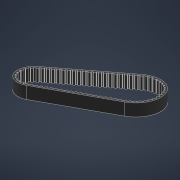
# Autodesk Inventor part: Parametric GT2 Belt v1
Saved by Autodesk Inventor 2021 (Build 250183000, 183)
## iProperties
Created: 2020-06-05
Part Number: Parametric GT2 Belt v1
Material: Rubber
Document SubType Name: Modeling
Designer: Bryce
Density: 0.93 g/cm^3
Appearance: Rubber - Black
Author: Bryce
Autodesk Inventor part; units mm, degrees
ref_plane "YZ Plane" through (0, 0, 0) normal (1, 0, 0) x (0, 1, 0)
ref_plane "XY Plane" through (0, 0, 0) normal (0, 0, 1) x (1, 0, 0)
sketch "top teeth placement" plane through (0, 0, 0) normal (0, 1, 0) x (-1, 0, 0)
  arc A0 (1.0993, -11.4063) -> (1.0993, 11.4063) centre (0, 0) ccw construction
  line L0 (1.0993, -11.4063) -> (-58.0762, -17.1095) construction
  line L1 (1.0993, 11.4063) -> (-58.0762, 17.1095) construction
  arc A1 (-58.0762, 17.1095) -> (-58.0762, -17.1095) centre (-59.7252, 0) ccw construction
  arc A2 (1.0993, -11.4063) -> (4.014, -10.7331) centre (0, 0) ccw construction
  arc A3 (-61.6201, -17.084) -> (-58.0762, -17.1095) centre (-59.7252, 0) ccw construction
  arc A4 (-64.5579, -16.4954) -> (-61.6201, -17.084) centre (-59.7252, 0) ccw construction
  line L2 (1.0993, -11.4063) -> (0, 0) construction
  line L3 (0, 0) -> (4.014, -10.7331) construction
  line L4 (-61.6201, -17.084) -> (-59.7252, 0) construction
  line L5 (-59.7252, 0) -> (-64.5579, -16.4954) construction
  point P0 (-1.8869, -11.6941)
  point P1 (-4.873, -11.9819)
  point P2 (-7.8592, -12.2697)
  point P3 (-10.8454, -12.5575)
  point P4 (-13.8315, -12.8453)
  point P5 (-16.8177, -13.1331)
  point P6 (-1.0925, 11.6175)
  point P7 (-4.0787, 11.9053)
  point P8 (-19.8038, -13.4209)
  point P9 (-22.79, -13.7087)
  point P10 (-25.7762, -13.9965)
  point P11 (-28.7623, -14.2843)
  point P12 (-31.7485, -14.5721)
  point P13 (-34.7347, -14.8599)
  point P14 (-37.7208, -15.1477)
  point P15 (-40.707, -15.4355)
  point P16 (-43.6931, -15.7233)
  point P17 (-46.6793, -16.0111)
  point P18 (-49.6655, -16.2989)
  point P19 (-52.6516, -16.5867)
  point P20 (-55.6378, -16.8745)
  point P21 (-58.624, -17.1622)
  dimension "pitch" = 3
  dimension "r_d35" = 60
  dimension "r_d36" = 33
  dimension "d17" = 22.9183
  dimension "d18" = 34.3775
  dimension "d30" = 3
  dimension "d35" = 59.4497
  dimension "d36" = 33.798
  dimension "d39" = 15
  dimension "d41" = 3
  dimension "d44" = 3.5503
  dimension "d45" = 57.303
  dimension "d48" = 10
  dimension "d50" = 3
  dimension "d52" = 2.202
  dimension "d62" = 3
  dimension "d71" = 59.7252
  constraints: 12 end point, 11 point on circle, 5 centre point, 4 coincident, 4 tangent, 3 concentric, 1 horizontal alignment, 1 point on line, 27 other
  measures "d17" diameter of A0
  measures "d18" diameter of A1
  measures "d30" distance of L2.start point (-1.887, -11.694)
  measures "d35" distance of L0.start L0.end
  measures "d52" distance of point (-1.093, 11.618) L1.start
  measures "d62" distance of point (-1.093, 11.618) point (-4.079, 11.905)
  measures "d71" distance of A1.centre point (0, 0)
sketch "gt2 profile" plane through (0, 0, 0) normal (0, 1, 0) x (-1, 0, 0)
  line L0 (-61.6201, -17.084) -> (-59.7252, 0) construction
  arc A0 (-58.0762, 17.1095) -> (-58.0762, -17.1095) centre (-59.7252, 0) ccw construction
  line L1 (1.0993, -11.4063) -> (-58.0762, -17.1095) construction
  line L2 (1.0993, 11.4063) -> (-58.0762, 17.1095) construction
  arc A1 (1.787, -10.3422) -> (0.2211, -10.4931) centre (1.0349, -10.7384) ccw
  arc A2 (1.9264, -10.723) -> (2.1945, -10.918) centre (2.1705, -10.6691) ccw
  line L3 (2.1945, -10.918) -> (-0.069, -11.1361)
  line L4 (0.4422, -11.0507) -> (1.0593, -10.9912) construction
  arc A3 (1.9264, -10.723) -> (1.787, -10.3422) centre (0.4422, -11.0507) ccw
  arc A4 (-0.069, -11.1361) -> (0.1569, -10.8936) centre (-0.093, -10.8873) ccw
  arc A5 (0.2211, -10.4931) -> (0.1569, -10.8936) centre (1.6764, -10.9317) ccw
  line L5 (2.2905, -11.9134) -> (0.0269, -12.1315)
  line L6 (2.2905, -11.9134) -> (2.1945, -10.918)
  line L7 (0.0269, -12.1315) -> (-0.069, -11.1361)
  line L8 (0.9534, -9.8923) -> (1.0628, -11.0271) construction
  line L9 (1.0593, -10.9912) -> (1.6764, -10.9317) construction
  arc A6 (-1.9708, 10.7044) -> (-0.4049, 10.5535) centre (-1.1569, 10.9496) ccw
  arc A7 (-2.0349, 11.1048) -> (-2.2609, 11.3474) centre (-2.2848, 11.0985) ccw
  line L10 (-2.2609, 11.3474) -> (0.0027, 11.1292)
  line L11 (-0.5154, 11.143) -> (-1.1325, 11.2024) construction
  arc A8 (-2.0349, 11.1048) -> (-1.9708, 10.7044) centre (-0.5154, 11.143) ccw
  arc A9 (0.0027, 11.1292) -> (-0.2654, 10.9343) centre (-0.0213, 10.8804) ccw
  arc A10 (-0.4049, 10.5535) -> (-0.2654, 10.9343) centre (-1.7497, 11.2619) ccw
  line L12 (-2.1649, 12.3428) -> (0.0986, 12.1246)
  line L13 (-2.1649, 12.3428) -> (-2.2609, 11.3474)
  line L14 (0.0986, 12.1246) -> (0.0027, 11.1292)
  line L15 (-1.2384, 10.1036) -> (-1.1291, 11.2383) construction
  line L16 (-1.1325, 11.2024) -> (-1.7497, 11.2619) construction
  arc A11 (-60.7288, -16.1835) -> (-62.2924, -16.0101) centre (-61.5461, -16.4171) ccw
  arc A12 (-60.6704, -16.5848) -> (-60.448, -16.8306) centre (-60.4205, -16.5822) ccw
  line L17 (-60.448, -16.8306) -> (-62.7082, -16.5799)
  line L18 (-62.1904, -16.6011) -> (-61.5741, -16.6695) construction
  arc A13 (-60.6704, -16.5848) -> (-60.7288, -16.1835) centre (-62.1904, -16.6011) ccw
  arc A14 (-62.7082, -16.5799) -> (-62.4373, -16.3889) centre (-62.6806, -16.3315) ccw
  arc A15 (-62.2924, -16.0101) -> (-62.4373, -16.3889) centre (-60.9579, -16.7378) ccw
  line L19 (-60.5583, -17.8245) -> (-62.8184, -17.5738)
  line L20 (-60.5583, -17.8245) -> (-60.448, -16.8306)
  line L21 (-62.8184, -17.5738) -> (-62.7082, -16.5799)
  line L22 (-61.4524, -15.5722) -> (-61.5781, -16.7053) construction
  line L23 (-61.5741, -16.6695) -> (-60.9579, -16.7378) construction
  line L24 (-61.3812, -17.1105) -> (-61.859, -17.0575) construction
  dimension "d170" = 0.85
  dimension "d172" = 0.25
  dimension "d173" = 0.381
  dimension "d175" = 0.62
  dimension "d176" = 1.52
  dimension "d177" = 1
  dimension "d178" = 1.14
  dimension "d185" = 0.85
  dimension "d186" = 0.25
  dimension "d187" = 0.62
  dimension "d188" = 1.52
  dimension "d189" = 1
  dimension "d190" = 1.14
  dimension "d192" = 0.381
  dimension "d193" = 2.202
  dimension "d194" = 0.85
  dimension "d195" = 0.25
  dimension "d196" = 0.62
  dimension "d197" = 1.52
  dimension "d198" = 1
  dimension "d199" = 1.14
  dimension "d200" = 0.381
  constraints: 44 end point, 33 point on circle, 19 tangent, 15 centre point, 13 perpendicular, 8 point on line, 5 parallel, 4 midpoint, 3 collinear, 3 equal radius
  measures "d170" radius of A1
  measures "d172" radius of A2
  measures "d173" distance between parallel lines of L1 L3
  measures "d175" distance of L4.start L4.end
  measures "d176" radius of A3
  measures "d177" distance between parallel lines of L5 L3
  measures "d178" distance of L8.start L8.end
  measures "d185" radius of A6
  measures "d186" radius of A7
  measures "d187" distance of L11.start L16.start
  measures "d188" radius of A8
  measures "d189" distance between parallel lines of L12 L10
  measures "d190" distance of L15.start L15.end
  measures "d192" distance between parallel lines of L2 L10
  measures "d193" distance from line of L2.start L15
  measures "d194" radius of A11
  measures "d195" radius of A12
  measures "d196" distance of L18.start L23.start
  measures "d197" radius of A13
  measures "d198" distance between parallel lines of L19 L17
  measures "d199" distance of L22.start L22.end
  measures "d200" distance between parallel lines of L24 L17
extrude "Top/Left Base Tooth" add sketch "gt2 profile" against normal mid plane 9 contours A3 A2 L3 A4 A5 A1 | L6 L5 L7 L3
pattern_sketch "Top Teeth" of "Top/Left Base Tooth" from (-1.0993, 0, -11.4063) copies at (1.8869, 0, -11.6941) at (4.873, 0, -11.9819) at (7.8592, 0, -12.2697) at (10.8454, 0, -12.5575) at (13.8315, 0, -12.8453) at (16.8177, 0, -13.1331) at (19.8038, 0, -13.4209) at (22.79, 0, -13.7087) at (25.7762, 0, -13.9965) at (28.7623, 0, -14.2843) at (31.7485, 0, -14.5721) at (34.7347, 0, -14.8599) at (37.7208, 0, -15.1477) at (40.707, 0, -15.4355) at (43.6931, 0, -15.7233) at (46.6793, 0, -16.0111) at (49.6655, 0, -16.2989) at (52.6516, 0, -16.5867) at (55.6378, 0, -16.8745) at (58.624, 0, -17.1622)
pattern_circular "Left Teeth" count 11 over 165 about axis through (0, 0, 0) along (0, 1, 0) of "Top/Left Base Tooth"
extrude "Right Base Tooth" add sketch "gt2 profile" along normal mid plane 9 contours A13 A12 L17 A14 A15 A11 | L20 L19 L21 L17
pattern_circular "Right Teeth" count 19 over 180 about axis through (59.7252, 0, 0) along (0, -1, 0) of "Right Base Tooth"
sketch "bottom teeth placement" plane through (0, 0, 0) normal (0, 1, 0) x (-1, 0, 0)
  arc A0 (1.0993, -11.4063) -> (1.0993, 11.4063) centre (0, 0) ccw construction
  line L0 (1.0993, -11.4063) -> (-58.0762, -17.1095) construction
  line L1 (1.0993, 11.4063) -> (-58.0762, 17.1095) construction
  arc A1 (-58.0762, 17.1095) -> (-58.0762, -17.1095) centre (-59.7252, 0) ccw construction
  point P0 (-1.0925, 11.6175)
  point P1 (-4.0787, 11.9053)
  point P2 (-7.0649, 12.1931)
  point P3 (-10.051, 12.4809)
  point P4 (-13.0372, 12.7687)
  point P5 (-16.0234, 13.0565)
  point P6 (-19.0095, 13.3443)
  point P7 (-21.9957, 13.6321)
  point P8 (-24.9818, 13.9199)
  point P9 (-27.968, 14.2077)
  point P10 (-30.9542, 14.4955)
  point P11 (-33.9403, 14.7833)
  point P12 (-36.9265, 15.0711)
  point P13 (-39.9127, 15.3589)
  point P14 (-42.8988, 15.6467)
  point P15 (-45.885, 15.9345)
  point P16 (-48.8712, 16.2223)
  point P17 (-51.8573, 16.5101)
  point P18 (-54.8435, 16.7979)
  point P19 (-57.8296, 17.0857)
  dimension "d144" = 3
  dimension "d147" = 33
  dimension "pitch" = 3
  dimension "d123" = 22.9183
  dimension "d124" = 34.3775
  dimension "d126" = 59.4497
  dimension "d127" = 33.798
  dimension "d131" = 57.303
  dimension "d134" = 2.202
  dimension "d135" = 3
  dimension "d136" = 59.7252
  constraints: 4 end point, 4 point on circle, 4 tangent, 2 centre point, 2 coincident, 1 horizontal alignment, 1 point on line, 20 other
  measures "d123" diameter of A0
  measures "d124" diameter of A1
  measures "d126" distance of L0.start L0.end
  measures "d134" distance of point (-1.093, 11.618) L1.start
  measures "d135" distance of point (-1.093, 11.618) point (-4.079, 11.905)
  measures "d136" distance of A1.centre point (0, 0)
extrude "Bottom Base Tooth" add sketch "gt2 profile" along normal mid plane 9 contours A8 A7 L10 A9 A10 A6 | L13 L12 L14 L10
pattern_sketch "Bottom Teeth" of "Bottom Base Tooth" from (1.0925, 0, 11.6175) copies at (4.0787, 0, 11.9053) at (7.0649, 0, 12.1931) at (10.051, 0, 12.4809) at (13.0372, 0, 12.7687) at (16.0234, 0, 13.0565) at (19.0095, 0, 13.3443) at (21.9957, 0, 13.6321) at (24.9818, 0, 13.9199) at (27.968, 0, 14.2077) at (30.9542, 0, 14.4955) at (33.9403, 0, 14.7833) at (36.9265, 0, 15.0711) at (39.9127, 0, 15.3589) at (42.8988, 0, 15.6467) at (45.885, 0, 15.9345) at (48.8712, 0, 16.2223) at (51.8573, 0, 16.5101) at (54.8435, 0, 16.7979) at (57.8296, 0, 17.0857)
sketch "Sketch8" plane through (0, 0, 0) normal (0, 1, 0) x (-1, 0, 0)
  arc A0 (1.0993, -11.4063) -> (1.0993, 11.4063) centre (0, 0) ccw construction
  line L0 (1.0993, -11.4063) -> (-58.0762, -17.1095) construction
  line L1 (1.0993, 11.4063) -> (-58.0762, 17.1095) construction
  arc A1 (-58.0762, 17.1095) -> (-58.0762, -17.1095) centre (-59.7252, 0) ccw construction
  arc A2 (1.1836, -12.2813) -> (1.1836, 12.2813) centre (0, 0) ccw
  line L2 (1.1836, -12.2813) -> (-57.9919, -17.9844)
  arc A3 (-57.9919, 17.9844) -> (-57.9919, -17.9844) centre (-59.7252, 0) ccw
  line L3 (-57.9919, 17.9844) -> (1.1836, 12.2813)
  arc A4 (1.0628, -11.0271) -> (1.0628, 11.0271) centre (0, 0) ccw
  line L4 (1.0628, -11.0271) -> (-58.1128, -16.7302)
  arc A5 (-58.1128, 16.7302) -> (-58.1128, -16.7302) centre (-59.7252, 0) ccw
  line L5 (-58.1128, 16.7302) -> (1.0628, 11.0271)
  dimension "d201" = 0.381
  dimension "d202" = 1.26
  constraints: 8 end point, 8 point on circle, 4 centre point, 6 other
  measures "d201" radial gap between concentric circles of A0 A4
  measures "d202" distance between parallel lines of L2 L4
extrude "Extrusion7" add sketch "Sketch8" along normal mid plane 9
equation "\"pitch\" = 3"
equation "\"r_d36\" = 33"
equation "\"d30\" = pitch"
equation "\"d41\" = pitch"
equation "\"d44\" = pitch + r_d35 - d35"
equation "\"d50\" = pitch"
equation "\"d62\" = pitch"
equation "\"d144\" = 3"
equation "\"d147\" = 33"
equation "\"r_d45\" = 57"
equation "\"pulley_1_angle\" = 15deg"
equation "\"pulley_2_angle\" = 10deg"
equation "\"d108\" = 5"
equation "\"d156\" = 5"
equation "\"center_distance\" = 59.72517"
equation "\"f_d35\" = 57"
equation "\"gt2_pld\" = 0.381"
equation "\"missing_tooth_bottom_right_round\" = 0"
equation "\"missing_tooth_bottom_right_straight\" = 0"
equation "\"missing_tooth_bottom_left\" = 0"
equation "\"belt_width\" = 9"
body "Solid3"
